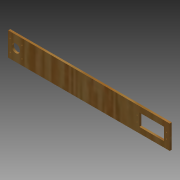
# Autodesk Inventor part: segment2b
Saved by Autodesk Inventor 2013 (Build 170138000, 138)
## iProperties
Created: 2014-10-09
Part Number: segment2b
Material: Plywood, Finish
Document SubType Name: Modeling
Designer: Masta
Density: 0.552 g/cm^3
Mass: 32.6528 g
Surface Area: 247.953 cm^2
Volume: 59.1536 cm^3
Author: Masta
Autodesk Inventor part; units mm, degrees
ref_plane "YZ Plane" through (0, 0, 0) normal (1, 0, 0) x (0, 1, 0)
ref_plane "XZ Plane" through (0, 0, 0) normal (0, 1, 0) x (-1, 0, 0)
ref_plane "XY Plane" through (0, 0, 0) normal (0, 0, 1) x (1, 0, 0)
sketch "Sketch1" plane through (0, 0, 0) normal (0, 1, 0) x (-1, 0, 0)
  line L0 (0, 0) -> (31.5, 0)
  line L1 (0, 0) -> (18.5, 0) construction
  line L2 (0, 0) -> (-10.5, 0)
  line L3 (-20, 0) -> (-20, 20)
  line L4 (-20, 20) -> (253, 20)
  line L5 (253, 20) -> (253, 0)
  line L6 (-10.5, 10.5) -> (31.5, 10.5)
  line L7 (31.5, 10.5) -> (31.5, -10.5)
  line L8 (31.5, -10.5) -> (-10.5, -10.5)
  line L9 (-10.5, -10.5) -> (-10.5, 10.5)
  line L10 (-10.5, 10.5) -> (31.5, -10.5) construction
  line L11 (31.5, 10.5) -> (-10.5, -10.5) construction
  line L12 (-14.5, 5) -> (35.5, 5) construction
  line L13 (35.5, 5) -> (35.5, -5) construction
  line L14 (35.5, -5) -> (-14.5, -5) construction
  line L15 (-14.5, -5) -> (-14.5, 5) construction
  line L16 (-14.5, 5) -> (35.5, -5) construction
  line L17 (35.5, 5) -> (-14.5, -5) construction
  line L18 (31.5, 0) -> (253, 0)
  line L19 (-10.5, 0) -> (-20, 0)
  line L20 (-20, 0) -> (0, 0) construction
  line L21 (240, 0) -> (240, 10) construction
  line L22 (240, 10) -> (250, 10) construction
  point P0 (10.5, 0)
  point P1 (10.5, 0)
  dimension "d28" = 18.5
  dimension "d37" = 20
  dimension "d38" = 20
  dimension "d39" = 42
  dimension "d40" = 21
  dimension "d41" = 50
  dimension "d42" = 10
  dimension "d43" = 10.5
  dimension "d52" = 240
  dimension "d53" = 13
  dimension "d54" = 9.5
  dimension "d62" = 10
  constraints: 46 end point, 8 perpendicular, 7 midpoint, 5 parallel, 4 coincident, 4 horizontal, 3 point on line, 1 collinear
  measures "d28" distance of L0.start L1.end
  measures "d37" distance of L5.end L4.end
  measures "d38" distance of L3.start L3.end
  measures "d39" distance of L7.end L8.end
  measures "d40" distance of L6.end L7.end
  measures "d41" distance of L13.end L14.end
  measures "d42" distance of L12.end L13.end
  measures "d43" distance from line of L9 point (0, 0)
  measures "d52" distance of L21.start point (0, 0)
  measures "d53" distance from line of L5 L21.start
  measures "d54" distance of L2.end L3.start
  measures "d62" distance of L21.start L21.end
extrude "Extrusion1" add sketch "Sketch1" along normal blind 3.5 contours L7 L6 L9 L19 L3 L4 L5 L18
hole "Hole3" at (0, 0, 0) at (14.5, 0, 5) at (-35.5, 0, 5) direction (0, 1, 0) diameter 2 end through all
fillet "Fillet1" [suppressed]
mirror "Mirror1" about plane through (-31.5, 0, 0) normal (0, 0, -1)
hole "Hole4" at (-240, 0, 0) direction (0, 1, 0) diameter 14 end through all
hole "Hole5" at (-250, 0, 10) direction (0, 1, 0) diameter 2 end through all
pattern_circular "Circular Pattern1" count 4 over 360 about axis through (-240, 275.937, 0) along (0, 1, 0) of "Hole5"
body "Solid1"
